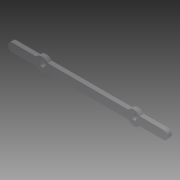
# Autodesk Inventor part: Handle
Saved by Autodesk Inventor 2015 (Build 190159000, 159)
## iProperties
Created: 2016-10-14
Part Number: Handle
Material: Generic
Document SubType Name: Modeling
Designer: James Yelland
Density: 1 g/cm^3
Appearance: Default
Author: James Yelland
Autodesk Inventor part; units mm, degrees
ref_plane "YZ Plane" through (0, 0, 0) normal (1, 0, 0) x (0, 1, 0)
ref_plane "XZ Plane" through (0, 0, 0) normal (0, 1, 0) x (-1, 0, 0)
ref_plane "XY Plane" through (0, 0, 0) normal (0, 0, 1) x (1, 0, 0)
sketch "Sketch1" plane through (0, 0, 0) normal (0, 1, 0) x (-1, 0, 0)
  circle A0 centre (-32.6132, 75.9327) radius 1.6
  circle A1 centre (32.6132, 75.9327) radius 1.6
  circle A2 centre (32.6132, 75.9327) radius 5
  circle A3 centre (-32.6132, 75.9327) radius 5
  line L0 (28.6132, 78.9327) -> (-28.6132, 78.9327)
  line L1 (-28.6132, 72.9327) -> (28.6132, 72.9327)
  line L2 (-28.6132, 72.9327) -> (28.6132, 72.9327) construction
  line L3 (36.6132, 72.9327) -> (53.6132, 72.9327)
  line L4 (36.6132, 72.9327) -> (53.6132, 72.9327) construction
  line L5 (56.6132, 75.9327) -> (56.6132, 75.9327)
  line L6 (53.6132, 78.9327) -> (36.6132, 78.9327)
  arc A4 (53.6132, 72.9327) -> (56.6132, 75.9327) centre (53.6132, 75.9327) ccw
  arc A5 (56.6132, 75.9327) -> (53.6132, 78.9327) centre (53.6132, 75.9327) ccw
  line L7 (-53.6132, 78.9327) -> (-36.6132, 78.9327)
  arc A6 (-53.6132, 78.9327) -> (-56.6132, 75.9327) centre (-53.6132, 75.9327) ccw
  arc A7 (-56.6132, 75.9327) -> (-53.6132, 72.9327) centre (-53.6132, 75.9327) ccw
  line L8 (-53.6132, 75.9327) -> (-53.6132, 72.9327) construction
  line L9 (-53.6132, 75.9327) -> (-56.6132, 75.9327) construction
  line L10 (-53.6132, 72.9327) -> (-36.6132, 72.9327)
  point P0 (0, 0)
  point P1 (36.6132, 78.9327)
  point P2 (56.6132, 72.9327)
  point P3 (56.6132, 78.9327)
  point P4 (-56.6132, 78.9327)
  dimension "d25" = 3.2
  dimension "d26" = 10
  dimension "d30" = 20
  dimension "d31" = 0
  dimension "d32" = 6
  dimension "d33" = 3
  dimension "d41" = 90
  constraints: 22 end point, 17 point on circle, 8 centre point, 5 horizontal, 5 point on line, 5 tangent, 3 coincident, 2 collinear, 1 concentric, 1 perpendicular
  measures "d25" diameter of A1
  measures "d26" diameter of A2
  measures "d30" distance of L3.start point (56.613, 72.933)
  measures "d31" distance between parallel lines of L3 L4
  measures "d32" distance of point (56.613, 72.933) point (56.613, 78.933)
  measures "d33" radius of A4
  measures "d41" angle of L9 L8
extrude "Extrusion1" add sketch "Sketch1" along normal blind 3
body "Solid1"
